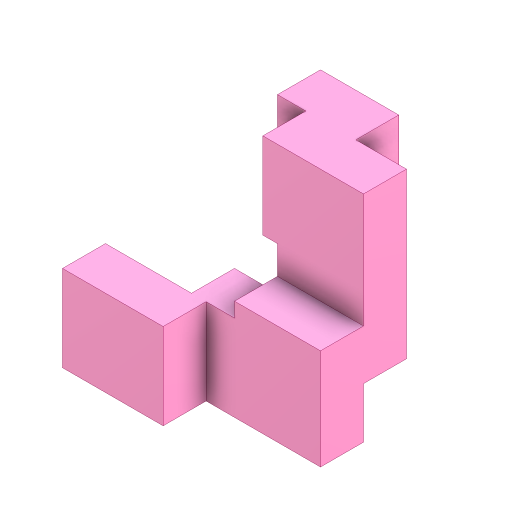
# Autodesk Inventor part: Template_ladder_2
Saved by Autodesk Inventor 2024 (Build 280153000, 153)
## iProperties
Created: 2023-03-18
Part Number: Template_ladder_2
Material: 一般
Document SubType Name: Modeling
Designer: USER
Density: 1 g/cm^3
Appearance: 平滑 - 紅色
Author: USER
Autodesk Inventor part; units mm, degrees
ref_plane "YZ Plane" through (0, 0, 0) normal (1, 0, 0) x (0, 1, 0)
ref_plane "XZ Plane" through (0, 0, 0) normal (0, 1, 0) x (-1, 0, 0)
ref_plane "XY Plane" through (0, 0, 0) normal (0, 0, 1) x (1, 0, 0)
sketch "草圖15" plane through (0, 0, 0) normal (0, 0, 1) x (1, 0, 0)
  line L0 (5, -5) -> (-5, -5)
  line L1 (-5, -5) -> (-5, 5)
  line L2 (-5, 5) -> (5, 5)
  line L3 (5, 5) -> (5, -5)
  line L4 (5, -5) -> (-5, 5) construction
  line L5 (-5, -5) -> (5, 5) construction
  line L6 (25, -25) -> (-25, -25)
  line L7 (-25, -25) -> (-25, 25)
  line L8 (-25, 25) -> (25, 25)
  line L9 (25, 25) -> (25, -25)
  line L10 (25, -25) -> (-25, 25) construction
  line L11 (-25, -25) -> (25, 25) construction
  line L12 (-25, -25) -> (-1.6, -25)
  line L13 (-1.6, -25) -> (-1.6, -5)
  line L14 (-1.6, -5) -> (-25, -5)
  line L15 (-25, -5) -> (-25, -25)
  line L16 (25, -25) -> (-1.6, -25)
  line L17 (-1.6, -5) -> (25, -5)
  line L18 (25, -5) -> (25, -25)
  line L19 (25, -25) -> (5, -25)
  line L20 (5, -25) -> (5, -1.6)
  line L21 (5, -1.6) -> (25, -1.6)
  line L22 (25, -1.6) -> (25, -25)
  line L23 (25, 25) -> (5, 25)
  line L24 (5, 25) -> (5, -1.6)
  line L25 (25, -1.6) -> (25, 25)
  line L26 (25, 25) -> (1.6, 25)
  line L27 (1.6, 25) -> (1.6, 5)
  line L28 (1.6, 5) -> (25, 5)
  line L29 (25, 5) -> (25, 25)
  line L30 (-25, 25) -> (1.6, 25)
  line L31 (1.6, 5) -> (-25, 5)
  line L32 (-25, 5) -> (-25, 25)
  line L33 (-5, -5) -> (-25, -5)
  line L34 (-25, -5) -> (-25, -25)
  line L35 (-25, -25) -> (-5, -25)
  line L36 (-5, -25) -> (-5, -5)
  line L37 (-1.6, -25) -> (-13.2, -25)
  line L38 (-13.2, -25) -> (-13.2, -5)
  line L39 (-13.2, -5) -> (-1.6, -5)
  line L40 (-1.6, -5) -> (-1.6, -25)
  line L41 (5, -1.6) -> (25, -1.6)
  line L42 (25, -1.6) -> (25, -13.2)
  line L43 (25, -13.2) -> (5, -13.2)
  line L44 (5, -13.2) -> (5, -1.6)
  line L45 (1.6, 5) -> (13.2, 5)
  line L46 (13.2, 5) -> (13.2, 25)
  line L47 (13.2, 25) -> (1.6, 25)
  line L48 (1.6, 25) -> (1.6, 5)
  line L49 (1.6, 5) -> (-5, 5)
  line L50 (-5, 5) -> (-5, 25)
  line L51 (-5, 25) -> (1.6, 25)
  line L52 (1.6, 25) -> (1.6, 5)
  point P0 (0, 0)
  point P1 (0, 0)
  point P2 (-1.6, -25)
  point P3 (-25, 5)
  point P4 (-5, 5)
  point P5 (-5, -25)
  point P6 (5, 5)
  point P7 (-5, -25)
  point P8 (-13.2, -25)
  point P9 (25, -13.2)
  point P10 (-5, 25)
  point P11 (-5, 5)
  point P12 (5, 5)
  point P13 (13.2, 5)
  point P14 (13.2, 25)
  dimension "d38" = 10
  dimension "d39" = 20
  dimension "d40" = 1.6
  dimension "d42" = 1.6
  dimension "d48" = 1.6
  dimension "d54" = 0
  dimension "d55" = 11.6
  dimension "d56" = 11.6
  dimension "d57" = 11.6
  dimension "d58" = 10
  constraints: 106 end point, 23 parallel, 13 horizontal, 13 perpendicular, 11 point on line, 4 midpoint, 1 coincident
  measures "d38" distance of L1.end L2.end
  measures "d39" distance between parallel lines of L8 L2
  measures "d40" distance from line of point (0, 0) L13
  measures "d42" distance from line of point (0, 0) L21
  measures "d48" distance from line of point (0, 0) L27
  measures "d54" distance between parallel lines of L7 L32
  measures "d55" distance between parallel lines of L38 L13
  measures "d56" distance between parallel lines of L41 L43
  measures "d57" distance between parallel lines of L27 L46
  measures "d58" distance between parallel lines of L50 L24
extrude "擠出10" add sketch "草圖15" against normal blind 10 contours L13 L6 L36 L0 | L36 L6 L38 L14 | L38 L6 L7 L14
extrude "擠出11" add sketch "草圖15" against normal blind 10 from surface at -10 contours L20 L6 L13 L0 | L3 L21 L9 L17 | L17 L9 L43 L20 | L13 L6 L36 L0 | L43 L9 L6 L20
extrude "擠出12" add sketch "草圖15" against normal blind 10 from surface at -20 contours L3 L21 L9 L17 | L17 L9 L43 L20 | L3 L28 L9 L21 | L2 L27 L8 L24 | L24 L8 L46 L28 | L46 L8 L9 L28
extrude "擠出13" add sketch "草圖15" against normal blind 10 from surface at -30 contours L2 L27 L8 L24 | L24 L8 L46 L28 | L50 L8 L27 L2
equation "\"d39\" = width"
equation "\"d40\" = gap"
equation "\"d42\" = gap"
equation "\"d48\" = gap"
equation "\"d55\" = stack"
equation "\"d56\" = stack"
equation "\"d57\" = stack"
equation "\"d44\" = height"
equation "\"d46\" = height"
equation "\"d50\" = height"
equation "\"d52\" = height"
equation "\"width\" = 20"
equation "\"height\" = 10"
equation "\"gap\" = 1.6"
equation "\"stack\" = 11.6"
